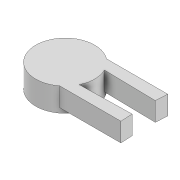
# Autodesk Inventor part: ab
Saved by Autodesk Inventor 2021 (Build 250183000, 183)
## iProperties
Created: 2021-07-07
Part Number: ab
Material: Generic
Document SubType Name: Modeling
Designer: Shaheen Khan
Density: 1 g/cm^3
Appearance: Default
Author: Shaheen Khan
Autodesk Inventor part; units mm, degrees
ref_plane "YZ Plane" through (0, 0, 0) normal (1, 0, 0) x (0, 1, 0)
ref_plane "XZ Plane" through (0, 0, 0) normal (0, 1, 0) x (-1, 0, 0)
ref_plane "XY Plane" through (0, 0, 0) normal (0, 0, 1) x (1, 0, 0)
sketch "Sketch1" plane through (0, 0, 0) normal (0, 1, 0) x (-1, 0, 0)
  circle A0 centre (0, 0) radius 12.5
  circle A1 centre (0, 0) radius 10
  circle A2 centre (0, 0) radius 9
  dimension "d0" = 25
  dimension "d1" = 20
  dimension "d2" = 18
  constraints: 3 centre point, 3 coincident
  measures "d0" diameter of A0
  measures "d1" diameter of A1
  measures "d2" diameter of A2
extrude "Extrusion1" add sketch "Sketch1" along normal blind 10 contours A0
sketch "Sketch2" plane through (0, 10, 0) normal (0, 1, 0) x (1, 0, 0)
  circle A0 centre (0, 0) radius 10
  circle A1 centre (0, 0) radius 9
  dimension "d5" = 18
  constraints: 2 centre point, 2 coincident
  measures "d5" diameter of A1
extrude "Extrusion2" add sketch "Sketch2" against normal blind 10 contours A0 | A1
sketch "Sketch3" plane through (0, 0, 0) normal (0, -1, 0) x (1, 0, 0)
  circle A0 centre (0, 0) radius 10
  circle A1 centre (0, 0) radius 9
  dimension "d8" = 20
  dimension "d9" = 18
  constraints: 2 centre point, 2 coincident
  measures "d8" diameter of A0
  measures "d9" diameter of A1
extrude "Extrusion3" cut sketch "Sketch3" against normal blind 5
sketch "Sketch4" plane through (0, 0, 0) normal (0, -1, 0) x (1, 0, 0)
  circle A0 centre (0, 0) radius 9 projected
  line L0 (-6.5324, -6.191) -> (-6.5324, 6.191)
  line L1 (-4.9332, -7.0348) -> (-4.9332, 6.9906)
  arc A1 (-4.9332, 6.9906) -> (-6.5324, 6.191) centre (-4.9332, 4.9917) ccw
  arc A2 (-6.5324, -6.191) -> (-4.9332, -7.0348) centre (-4.9332, -5.0977) ccw
  point P0 (-6.1136, 6.6049)
  point P1 (-5.9735, -6.7318)
  constraints: 6 point on circle, 4 end point, 2 centre point, 2 point on line, 2 vertical
extrude "Extrusion4" cut sketch "Sketch4" against normal blind 5 contours A0 A1 L1 A2 L0
sketch "Sketch5" plane through (0, 0, 0) normal (0, -1, 0) x (1, 0, 0)
  arc A0 (-5.9735, -6.7318) -> (-6.1136, 6.6049) centre (0, 0) ccw projected
  line L0 (-1.1999, -8.9197) -> (-1.1999, 8.9197)
  line L1 (1.1999, 8.9197) -> (1.1999, -8.9197)
  line L2 (6.5028, 6.222) -> (6.5028, -5.7075)
  line L3 (6.5028, -5.7075) -> (5.4199, -6.7318)
  line L4 (5.4199, -6.7318) -> (5.4199, 7.185)
  constraints: 10 end point, 6 point on circle, 2 parallel, 2 vertical
extrude "Extrusion5" cut sketch "Sketch5" against normal blind 5 contours L0 A0 L1 | L2 L3 L4 A0
sketch "Sketch6" plane through (0, 10, 0) normal (0, 1, 0) x (1, 0, 0)
  circle A0 centre (0, 0) radius 12.5 projected
  line L0 (7.5517, 9.961) -> (33.5517, 9.961)
  line L1 (33.5517, 9.961) -> (33.2795, 4.9684)
  line L2 (33.2795, 4.9684) -> (11.2795, 5.3874)
  line L3 (13.1769, 0.0291) -> (33.0118, 0.0291)
  line L4 (7.5517, -9.9028) -> (33.5517, -9.9028)
  line L5 (33.5517, -9.9028) -> (33.2795, -4.9102)
  line L6 (33.2795, -4.9102) -> (11.2795, -5.3291)
  point P0 (11.3073, -5.3286)
  point P1 (7.6279, -9.9028)
  dimension "d16" = 26
  dimension "d17" = 5
  dimension "d18" = 22
  constraints: 14 end point, 4 symmetric about line, 2 horizontal, 2 point on circle
  measures "d16" distance of L0.start L0.end
  measures "d17" distance of L0.end L1.end
  measures "d18" horizontal distance of L1.end L2.end
extrude "Extrusion6" add sketch "Sketch6" against normal blind 8 contours A0 L0 L1 L2 | L6 L5 L4 A0
body "Solid1"
